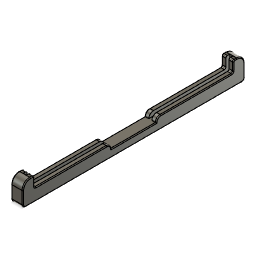
Hynix_DDR5_insertion_tool_v2 (Autodesk Fusion 360 design; units mm, degrees)
Autodesk Fusion 360 part; units mm, degrees
sketch "Sketch1" plane through (0, 0, 0) normal (0, 1, 0) x (1, 0, 0)
  line L0 (3.75, -72) -> (-3.75, -72)
  line L1 (-3.75, -72) -> (-3.75, 72)
  line L2 (-3.75, 72) -> (3.75, 72)
  line L3 (3.75, 72) -> (3.75, -72)
  line L4 (3.75, -72) -> (-3.75, 72) construction
  line L5 (-3.75, -72) -> (3.75, 72) construction
  dimension "d1" = 7.5
  dimension "d2" = 144
  constraint horizontal L0
  constraint perpendicular L0 L1
  constraint parallel L0 L2
  constraint parallel L1 L3
  constraint coincident L4 origin
  constraint coincident L5 origin
  measures "d1" distance of L1.end L2.end
  measures "d2" distance of L0.start L2.end
extrude "Extrude1" add sketch "Sketch1" along normal blind 5
sketch "Sketch2" plane through (0, 5, 0) normal (0, 1, 0) x (-1, 0, 0)
  line L0 (-3.75, -72) -> (3.75, -72)
  line L1 (3.75, -72) -> (3.75, 72)
  line L2 (3.75, 72) -> (-3.75, 72)
  line L3 (-3.75, 72) -> (-3.75, -72)
  line L4 (3.75, 72) -> (-3.75, 72)
  line L5 (-3.75, 72) -> (-3.75, 67)
  line L6 (-3.75, 67) -> (3.75, 67)
  line L7 (3.75, 67) -> (3.75, 72)
  dimension "d5" = 5
  constraint horizontal L4
  constraint vertical L5
  constraint horizontal L6
  constraint vertical L7
  constraint coincident L3 L5.end
  constraint coincident L1.end L2.start
  measures "d5" distance of L2.end L5.end
extrude "Extrude2" add sketch "Sketch2" along normal blind 10 contours L1 L2 L3 L4 L5 L6 L7
sketch "Sketch3" plane through (0, 5, 0) normal (0, 1, 0) x (-1, 0, 0)
  line L0 (3.75, 67) -> (-3.75, 67)
  line L1 (-3.75, 67) -> (-3.75, -72)
  line L2 (-3.75, -72) -> (3.75, -72)
  line L3 (3.75, -72) -> (3.75, 67)
  line L4 (3.75, -72) -> (-3.75, -72)
  line L5 (-3.75, -72) -> (-3.75, -67)
  line L6 (-3.75, -67) -> (3.75, -67)
  line L7 (3.75, -67) -> (3.75, -72)
  dimension "d8" = 5
  constraint horizontal L4
  constraint vertical L5
  constraint horizontal L6
  constraint vertical L7
  constraint coincident L1 L5.end
  constraint coincident L2.end L3.start
  measures "d8" distance of L1.end L5.end
extrude "Extrude3" add sketch "Sketch3" along normal blind 10 contours L1 L2 L3 L4 L5 L6 L7
fillet "Fillet1" radius 5 1 edges at (0, 15, 72)
fillet "Fillet2" radius 5 1 edges at (0, 15, -72)
sketch "Sketch6" plane through (0, 5, 0) normal (0, 1, 0) x (-1, 0, 0)
  line L0 (-3.75, -67) -> (3.75, -67)
  line L1 (3.75, -67) -> (3.75, 67)
  line L2 (3.75, 67) -> (-3.75, 67)
  line L3 (-3.75, 67) -> (-3.75, -67)
  line L4 (3.75, -67) -> (1, -67)
  line L5 (1, -67) -> (1, -64.5)
  line L6 (1, -64.5) -> (3.75, -64.5)
  line L7 (3.75, -64.5) -> (3.75, -67)
  line L8 (-3.75, -67) -> (-1, -67)
  line L9 (-1, -67) -> (-1, -64.5)
  line L10 (-1, -64.5) -> (-3.75, -64.5)
  line L11 (-3.75, -64.5) -> (-3.75, -67)
  dimension "d18" = 2.75
  dimension "d19" = 2.5
  dimension "d20" = 2.75
  dimension "d21" = 2.5
  constraint horizontal L4
  constraint vertical L5
  constraint horizontal L6
  constraint vertical L7
  constraint coincident L0.end L1.start
  constraint horizontal L8
  constraint vertical L9
  constraint horizontal L10
  constraint vertical L11
  constraint coincident L0.start L3.end
  measures "d18" distance of L0.end L4.end
  measures "d19" distance of L0.end L6.end
  measures "d20" distance of L0.start L8.end
  measures "d21" distance of L0.start L10.end
extrude "Extrude5" add sketch "Sketch6" along normal blind 10 contours L0 L3 L8 L9 L10 L11 | L0 L1 L4 L5 L6 L7
sketch "Sketch7" plane through (0, 5, 0) normal (0, 1, 0) x (-1, 0, 0)
  line L0 (1, -67) -> (1, -64.5)
  line L1 (1, -64.5) -> (3.75, -64.5)
  line L2 (3.75, -64.5) -> (3.75, 67)
  line L3 (3.75, 67) -> (-3.75, 67)
  line L4 (-3.75, 67) -> (-3.75, -64.5)
  line L5 (-3.75, -64.5) -> (-1, -64.5)
  line L6 (-1, -64.5) -> (-1, -67)
  line L7 (-1, -67) -> (1, -67)
  line L8 (-3.75, 67) -> (-1, 67)
  line L9 (-1, 67) -> (-1, 64.5)
  line L10 (-1, 64.5) -> (-3.75, 64.5)
  line L11 (-3.75, 64.5) -> (-3.75, 67)
  dimension "d24" = 2.75
  dimension "d25" = 2.5
  constraint horizontal L8
  constraint vertical L9
  constraint horizontal L10
  constraint vertical L11
  constraint coincident L3.end L4.start
  measures "d24" distance of L3.end L8.end
  measures "d25" distance of L3.end L10.end
sketch "Sketch8" plane through (0, 5, 0) normal (0, 1, 0) x (-1, 0, 0)
  line L0 (3.75, 67) -> (1, 67)
  line L1 (1, 67) -> (1, 64.5)
  line L2 (1, 64.5) -> (3.75, 64.5)
  line L3 (3.75, 64.5) -> (3.75, 67)
  point P0 (3.75, 67)
  dimension "d26" = 2.75
  dimension "d27" = 2.5
  constraint horizontal L0
  constraint vertical L1
  constraint horizontal L2
  constraint vertical L3
  constraint coincident P0 L0.start
  measures "d26" distance of P0 L0.end
  measures "d27" distance of P0 L2.end
extrude "Extrude6" add sketch "Sketch8" sketch "Sketch7" along normal blind 10 of sketch 2 contours L3 L4 L8 L9 L10 L11
sketch "Sketch9" plane through (0, 5, 0) normal (0, 1, 0) x (-1, 0, 0)
  line L0 (-1, 67) -> (-1, 64.5)
  line L1 (-1, 64.5) -> (-3.75, 64.5)
  line L2 (-3.75, 64.5) -> (-3.75, -64.5)
  line L3 (-3.75, -64.5) -> (-1, -64.5)
  line L4 (-1, -64.5) -> (-1, -67)
  line L5 (-1, -67) -> (1, -67)
  line L6 (1, -67) -> (1, -64.5)
  line L7 (1, -64.5) -> (3.75, -64.5)
  line L8 (3.75, -64.5) -> (3.75, 64.5)
  line L9 (3.75, 64.5) -> (1, 64.5)
  line L10 (1, 64.5) -> (1, 67)
  line L11 (1, 67) -> (-1, 67)
  line L12 (-3.75, 64.5) -> (-1, 64.5)
  line L13 (-1, 64.5) -> (-1, 14.5)
  line L14 (-1, 14.5) -> (-3.75, 14.5)
  line L15 (-3.75, 14.5) -> (-3.75, 64.5)
  line L16 (3.75, 64.5) -> (1, 64.5)
  line L17 (1, 64.5) -> (1, 14.5)
  line L18 (1, 14.5) -> (3.75, 14.5)
  line L19 (3.75, 14.5) -> (3.75, 64.5)
  line L20 (3.75, -64.5) -> (1, -64.5)
  line L21 (1, -64.5) -> (1, -14.5)
  line L22 (1, -14.5) -> (3.75, -14.5)
  line L23 (3.75, -14.5) -> (3.75, -64.5)
  line L24 (-3.75, -64.5) -> (-1, -64.5)
  line L25 (-1, -64.5) -> (-1, -14.5)
  line L26 (-1, -14.5) -> (-3.75, -14.5)
  line L27 (-3.75, -14.5) -> (-3.75, -64.5)
  dimension "d30" = 2.75
  dimension "d31" = 50
  dimension "d32" = 2.75
  dimension "d33" = 50
  dimension "d34" = 2.75
  dimension "d35" = 50
  dimension "d36" = 2.75
  dimension "d37" = 50
  constraint horizontal L12
  constraint vertical L13
  constraint horizontal L14
  constraint vertical L15
  constraint coincident L1.end L2.start
  constraint horizontal L16
  constraint vertical L17
  constraint horizontal L18
  constraint vertical L19
  constraint coincident L8.end L9.start
  constraint horizontal L20
  constraint vertical L21
  constraint horizontal L22
  constraint vertical L23
  constraint coincident L7.end L8.start
  constraint horizontal L24
  constraint vertical L25
  constraint horizontal L26
  constraint vertical L27
  constraint coincident L2.end L3.start
  measures "d30" distance of L1.end L0.end
  measures "d31" distance of L1.end L14.end
  measures "d32" distance of L8.end L9.end
  measures "d33" distance of L8.end L18.end
  measures "d34" distance of L7.end L6.end
  measures "d35" distance of L7.end L22.end
  measures "d36" distance of L2.end L3.end
  measures "d37" distance of L2.end L26.end
extrude "Extrude7" add sketch "Sketch9" along normal blind 3 contours L1 L2 L12 L13 L14 L15 | L8 L9 L16 L17 L18 L19 | L2 L3 L24 L25 L26 L27 | L7 L8 L20 L21 L22 L23
fillet "Fillet3" radius 3 4 edges at (2.375, 8, -14.5) (-2.375, 8, -14.5) (-2.375, 8, 14.5) (2.375, 8, 14.5)
fillet "Fillet4" radius 1 4 edges at (-2.375, 15, 64.5) (2.375, 15, 64.5) (-2.375, 15, -64.5) (2.375, 15, -64.5)
fillet "Fillet5" radius 1 4 edges at (-2.375, 8, -64.5) (2.375, 8, -64.5) (2.375, 8, 64.5) (-2.375, 8, 64.5)
fillet "Fillet6" radius 2 1 edges at (0, 0, -72)
fillet "Fillet7" radius 2 1 edges at (0, 0, 72)
fillet "Fillet8" radius 0.5 20 edges at (-3.75, 7.1213, 15.3787) (-3.75, 8, 40.5) (-3.75, 8.2929, 64.2071) (-3.75, 11.5, 64.5) (-3.75, 14.7071, 64.7929) (-3.75, 15, 66.25) (-3.75, 13.5355, 70.5355) (-3.75, 6, 72) (-3.75, 0.5858, 71.4142) (-3.75, 0, 0) (-3.75, 0.5858, -71.4142) (-3.75, 6, -72) (-3.75, 13.5355, -70.5355) (-3.75, 15, -66.25) (-3.75, 14.7071, -64.7929) (-3.75, 11.5, -64.5) (-3.75, 8.2929, -64.2071) (-3.75, 8, -40.5) (-3.75, 7.1213, -15.3787) (-3.75, 5, 0)
fillet "Fillet9" radius 0.5 20 edges at (3.75, 7.1213, -15.3787) (3.75, 8, -40.5) (3.75, 8.2929, -64.2071) (3.75, 11.5, -64.5) (3.75, 14.7071, -64.7929) (3.75, 15, -66.25) (3.75, 13.5355, -70.5355) (3.75, 6, -72) (3.75, 0.5858, -71.4142) (3.75, 0, 0) (3.75, 0.5858, 71.4142) (3.75, 6, 72) (3.75, 13.5355, 70.5355) (3.75, 15, 66.25) (3.75, 14.7071, 64.7929) (3.75, 11.5, 64.5) (3.75, 8.2929, 64.2071) (3.75, 8, 40.5) (3.75, 7.1213, 15.3787) (3.75, 5, 0)
